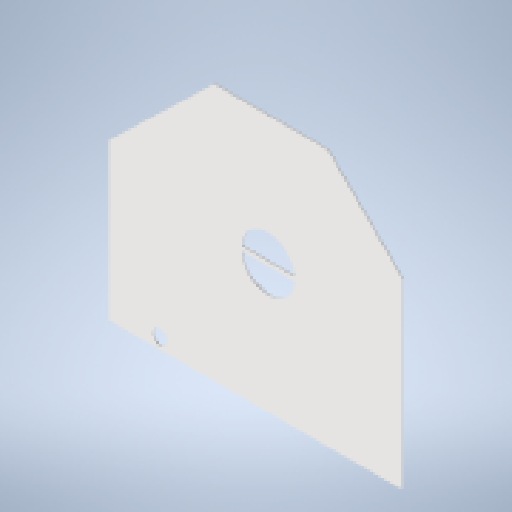
# Autodesk Inventor part: Left wall
Saved by Autodesk Inventor 2024.2 (Build 282272000, 272)
## iProperties
Created: 2023-08-31
Part Number: Left wall
Material: Generic
Document SubType Name: Modeling
Designer: admin
Density: 1 g/cm^3
Appearance: Default
Author: admin
Autodesk Inventor part; units mm, degrees
ref_plane "YZ Plane" through (0, 0, 0) normal (1, 0, 0) x (0, 1, 0)
ref_plane "XZ Plane" through (0, 0, 0) normal (0, 1, 0) x (-1, 0, 0)
ref_plane "XY Plane" through (0, 0, 0) normal (0, 0, 1) x (1, 0, 0)
sketch "Sketch1" plane through (0, 0, 0) normal (0, 0, 1) x (1, 0, 0)
  line L0 (0, 0) -> (0, 1900) construction
  line L1 (440, 1900) -> (-400, 1900)
  line L2 (-400, 1900) -> (-1180, 1150)
  line L3 (-1180, 0) -> (-1180, 1150)
  line L4 (990, 0) -> (990, 1350)
  line L5 (440, 1900) -> (990, 1350)
  circle A0 centre (0, 950) radius 250 construction
  line L6 (990, 0) -> (-1180, 0)
  circle A1 centre (-1701.6377, -269.2167) radius 188.5 construction
  circle A2 centre (-800, 80) radius 54
  circle A3 centre (0, 950) radius 200
  line L7 (0, 1200) -> (0, 1150) construction
  line L8 (-721.2646, 950) -> (721.2646, 950) construction
  line L9 (-200, 950) -> (-205, 950) construction
  line L10 (-205, 955) -> (-205, 945)
  line L11 (-205, 955) -> (-199.9375, 955)
  line L12 (-205, 945) -> (-199.9375, 945)
  line L13 (200, 950) -> (205, 950) construction
  line L14 (205, 955) -> (205, 945)
  line L15 (199.9375, 955) -> (205, 955)
  line L16 (205, 945) -> (199.9375, 945)
  line L17 (-205, 965) -> (205, 965)
  line L18 (205, 965) -> (205, 935)
  line L19 (205, 935) -> (-205, 935)
  line L20 (-205, 935) -> (-205, 965)
  line L21 (5, 1151.9375) -> (5, 1149.9375)
  line L22 (5, 1151.9375) -> (-5, 1151.9375)
  line L23 (-5, 1151.9375) -> (-5, 1149.9375)
  line L24 (5, 748.0625) -> (-5, 748.0625)
  line L25 (-5, 748.0625) -> (-5, 750.0625)
  line L26 (5, 748.0625) -> (5, 750.0625)
  point P0 (0, 950)
  point P1 (-199.4367, 935)
  point P2 (199.4367, 935)
  point P3 (199.4367, 965)
  point P4 (-199.4367, 965)
  point P5 (0, 1151.9375)
  dimension "d52" = 500
  dimension "d1" = 840
  dimension "d3" = 1150
  dimension "d8" = 45
  dimension "d9" = 1082.0813
  dimension "d10" = 550
  dimension "d12" = 1180
  dimension "d13" = 950
  dimension "d14" = 108
  dimension "d15" = 1900
  dimension "d17" = -521.6377
  dimension "d18" = 377
  dimension "d19" = -269.2167
  dimension "d34" = 380
  dimension "d35" = 80
  dimension "d37" = 2170
  dimension "d38" = 50
  dimension "d53" = 5
  dimension "d54" = 10
  dimension "d55" = 30
  dimension "d57" = 2
  dimension "d58" = 10
  constraints: 54 end point, 10 horizontal, 8 midpoint, 8 point on line, 7 vertical, 5 equal length, 3 perpendicular, 2 centre point, 2 parallel, 2 vertical alignment, 1 coincident, 15 other
  measures "d1" distance of L1.start L1.end
  measures "d3" distance of L3.start L2.end
  measures "d8" angle of L5 L4
  measures "d9" distance of L1.end L2.end
  measures "d10" distance from line of L4.end L1
  measures "d12" distance from line of L3 point (0, 950)
  measures "d13" distance from line of L6 point (0, 950)
  measures "d14" diameter of A2
  measures "d15" vertical distance of L3.start L1.end
  measures "d17" distance from line of L3 A1.centre
  measures "d18" diameter of A1
  measures "d19" distance from line of A1.centre L6
  measures "d34" distance from line of A2.centre L3
  measures "d35" distance from line of A2.centre L6
  measures "d37" distance between parallel lines of L4 L3
  measures "d38" distance of L7.start L7.end
  measures "d53" distance of L9.end L9.start
  measures "d54" distance of L10.start L10.end
  measures "d55" distance between parallel lines of L19 L17
  measures "d57" distance of L21.start L21.end
  measures "d58" distance of L21.start L22.end
extrude "Extrusion1" add sketch "Sketch1" along normal blind 10 contours L5 L4 L6 L3 L2 L1 | A3 L19 L17 | A3 L15 L14 L16 | A3 L17 L18 L15 | L16 L18 L19 A3 | A3 L11 L20 L17 | L19 L20 L12 A3 | A3 L12 L10 L11
fillet "Fillet1" radius 10 4 edges at (-199.4367, 965, 5) (-199.4367, 935, 5) (199.4367, 965, 5) (199.4367, 935, 5)
sketch "Sketch4" plane through (0, 0, 0) normal (0, 0, 1) x (1, 0, 0)
  circle A0 centre (-48.7726, 1195.1963) radius 9
  arc A1 (-5, 1149.9375) -> (-198.2611, 976.3158) centre (0, 950) ccw projected
  line L0 (0, 950) -> (0, 1196.7062) construction
  line L1 (-48.7726, 1195.1963) -> (0, 950) construction
  point P0 (0, 0)
  dimension "d59" = 250
  dimension "d60" = 18
  dimension "d61" = 11.25
  constraints: 4 end point, 1 centre point, 1 vertical
  measures "d59" distance of L0.start L1.start
  measures "d60" diameter of A0
  measures "d61" angle of L1 L0
extrude "Extrusion4" cut sketch "Sketch4" along normal blind 10
pattern_circular "Circular Pattern3" count 16 over 360 about axis through (0, 950, 0) along (0, 0, 1) of "Extrusion4"
equation "\"d8\" = d4"
equation "\"d4\" = 45deg"
body "Solid1"
